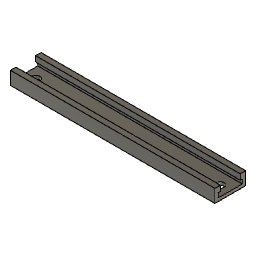
Alu_M6_M8_T-Track_Sliding_nut_T_100mm_holes_ext (Autodesk Fusion 360 design; units mm, degrees)
Autodesk Fusion 360 part; units mm, degrees
sketch "frame_ext_YZ" plane through (0, 0, 0) normal (1, 0, 0) x (0, 1, 0)
  line L0 (0, 0) -> (15, 0)
  line L1 (15, 0) -> (15, 12.8)
  line L2 (0, 0) -> (0, 15) construction
  line L3 (15, 12.8) -> (9.65, 12.8)
  line L4 (9.65, 12.8) -> (9.65, 7.4)
  line L5 (9.65, 7.4) -> (11.8, 7.4)
  line L6 (11.8, 7.4) -> (11.8, 3.1)
  line L7 (11.8, 3.1) -> (0, 3.1)
  line L8 (-9.65, 12.8) -> (-9.65, 7.4)
  line L9 (-9.65, 7.4) -> (-11.8, 7.4)
  line L10 (-11.8, 7.4) -> (-11.8, 3.1)
  line L11 (0, 0) -> (-15, 0)
  line L12 (-15, 12.8) -> (-9.65, 12.8)
  line L13 (-15, 0) -> (-15, 12.8)
  line L14 (-11.8, 3.1) -> (0, 3.1)
  dimension "d1" = 15
  dimension "d2" = 12.8
  dimension "d4" = 5.35
  dimension "d5" = 5.4
  dimension "d11" = 2.15
  dimension "d12" = 4.3
  constraint coincident L0.start L2.start
  constraint horizontal L0
  constraint perpendicular L0 L1
  constraint perpendicular L0 L2
  constraint perpendicular L1 L3
  constraint perpendicular L3 L4
  constraint perpendicular L4 L5
  constraint perpendicular L5 L6
  constraint coincident L2 L7.end
  constraint perpendicular L2 L7
  constraint symmetric L0.start L2 L11.start
  constraint symmetric L0.end L2 L11.end
  constraint symmetric L1.end L2 L12.start
  constraint symmetric L2 L3.end L8.start
  constraint symmetric L2 L4.end L8.end
  constraint symmetric L2 L5.end L9.end
  constraint symmetric L2 L6.end L10.end
  constraint symmetric L2 L7.end L14.end
  measures "d1" distance of L0.start L0.end
  measures "d2" distance of L0.end L1.end
  measures "d4" distance of L1.end L3.end
  measures "d5" distance of L3.end L4.end
  measures "d11" distance of L4.end L5.end
  measures "d12" distance of L5.end L6.end
extrude "Extrude1" add sketch "frame_ext_YZ" along normal mid plane 200
sketch "frame_ext_YX" plane through (0, 0, 3.1) normal (0, 0, 1) x (-1, 0, 0)
  line L0 (100, 11.8) -> (-100, 11.8)
  line L1 (-100, 11.8) -> (-100, -11.8)
  line L2 (-100, -11.8) -> (100, -11.8)
  line L3 (100, -11.8) -> (100, 11.8)
  line L4 (0, 0) -> (-90, 0) construction
  circle A0 centre (-90, 0) radius 4
  line L5 (0, 0) -> (0, 53.6768) construction
  circle A1 centre (90, 0) radius 4
  dimension "d16" = 90
  dimension "d17" = 8
  constraint coincident L4.start L5.start
  constraint parallel L2 L4
  constraint coincident L4.end A0.centre
  constraint perpendicular L4 L5
  constraint symmetric A0 L5 A1
  measures "d16" distance of L4.start L4.end
  measures "d17" diameter of A0
extrude "Extrude2" cut sketch "frame_ext_YX" against normal up to surface (3.1 mm away) contours A0 | A1
equation "d4 = ( 30 / 2 ) * 1 mm - ( 19.3 / 2 ) * 1 mm"
equation "Alu_M6_M8_T_track_length = 100 mm" comment "dlugosc ramki"
equation "d14 = Alu_M6_M8_T_track_length"
equation "d16 = Alu_M6_M8_T_track_length - 10 mm"
named bodies: "Alu_M6_M8_T-Track_Sliding_nut_T_100mm_holes_ext"
